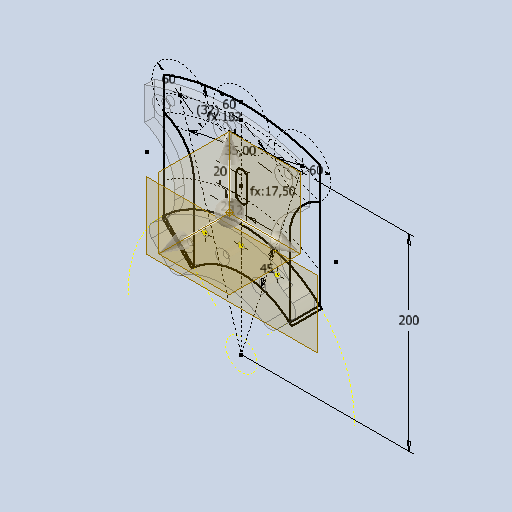
# Autodesk Inventor part: CounterweightFixation_Axis0
Saved by Autodesk Inventor 2024 (Build 280153000, 153)
## iProperties
Created: 2022-10-27
Part Number: CounterweightFixation_Axis0
Material: PMMA-Kunststoff
Document SubType Name: Modeling
Designer: alexw
Mass: 326.548 g
Surface Area: 547.419 cm^2
Volume: 274.872 cm^3
Density: 1.188 g/cm^3
Appearance: Polycarbonat - klar
Author: alexw
Autodesk Inventor part; units mm, degrees
ref_plane "YZ Plane" through (0, 0, 0) normal (1, 0, 0) x (0, 1, 0)
ref_plane "XZ Plane" through (0, 0, 0) normal (0, 1, 0) x (-1, 0, 0)
ref_plane "XY Plane" through (0, 0, 0) normal (0, 0, 1) x (1, 0, 0)
sketch "Skizze1" plane through (0, 0, 0) normal (0, 0, 1) x (1, 0, 0)
  arc A0 (119.8865, -45.2174) -> (-119.8865, -45.2174) centre (0, -40) ccw construction
  arc A1 (53.033, 13.033) -> (-53.033, 13.033) centre (0, -40) ccw construction
  line L0 (53.033, 13.033) -> (84.8528, 44.8528)
  line L1 (26.163, -9.5944) -> (68.5894, 32.832) construction
  line L2 (0, 0) -> (0, 80) construction
  line L3 (-53.033, 13.033) -> (-84.8528, 44.8528)
  arc A2 (53.033, 13.033) -> (-53.033, 13.033) centre (0, -40) ccw
  arc A3 (84.8528, 44.8528) -> (-84.8528, 44.8528) centre (0, -40) ccw
  arc A4 (41.04, 51.2399) -> (35.4967, 53.536) centre (38.2683, 52.388) ccw construction
  arc A5 (-35.4967, 53.536) -> (-41.04, 51.2399) centre (-38.2683, 52.388) ccw construction
  arc A6 (3, 60) -> (-3, 60) centre (0, 60) ccw construction
  line L4 (50.8692, 15.1119) -> (82.705, 46.9476)
  line L5 (-68.5894, 32.832) -> (-26.163, -9.5944) construction
  line L6 (-50.8692, 15.1119) -> (-82.705, 46.9476)
  circle A7 centre (0, -40) radius 16.5 construction
  line L7 (0, -40) -> (0, 160) construction
  arc A8 (82.705, 176.7577) -> (-82.705, 176.7577) centre (0, -40) ccw
  line L8 (82.705, 46.9476) -> (82.705, 176.7577)
  line L9 (-82.705, 46.9476) -> (-82.705, 176.7577)
  arc A9 (82.705, 142.0986) -> (-82.705, 142.0986) centre (0, -40) ccw construction
  line L10 (50.8692, 15.1119) -> (50.8692, 95.7841)
  arc A10 (82.705, 142.0986) -> (50.8692, 95.7841) centre (100.4762, 95.7841) ccw
  arc A11 (82.705, 79.1003) -> (-82.705, 79.1003) centre (0, -40) ccw construction
  line L11 (-50.8692, 15.1119) -> (-50.8692, 95.7841)
  arc A12 (-50.8692, 95.7841) -> (-82.705, 142.0986) centre (-100.4762, 95.7841) ccw
  arc A13 (82.705, 159.5392) -> (-82.705, 159.5392) centre (0, -40) ccw construction
  line L12 (64.9525, 166.0029) -> (0, -40) construction
  line L13 (0, -40) -> (-64.9525, 166.0029) construction
  circle A14 centre (64.9525, 166.0029) radius 30 construction
  circle A15 centre (0, 176) radius 30 construction
  circle A16 centre (-64.9525, 166.0029) radius 30 construction
  line L14 (0, 105) -> (0, 125) construction
  line L15 (6, 105) -> (6, 125)
  line L16 (-6, 125) -> (-6, 105)
  arc A17 (-6, 105) -> (6, 105) centre (0, 105) ccw
  arc A18 (6, 125) -> (-6, 125) centre (0, 125) ccw
  point P0 (0, 192)
  point P1 (-50.8692, 68.6845)
  point P2 (50.8692, 68.6845)
  point P3 (0, 115)
  dimension "d0" = 45
  dimension "d4" = 200
  dimension "d5" = 32
  dimension "d6" = 25
  dimension "d7" = 32
  dimension "d8" = 16
  dimension "d9" = 35
  dimension "d10" = 17.5
  dimension "d11" = 60
  dimension "d12" = 60
  dimension "d13" = 60
  dimension "d32" = 20
  dimension "d33" = 12
  constraints: 37 point on circle, 32 end point, 14 centre point, 11 point on line, 8 coincident, 6 tangent, 4 concentric, 4 symmetric about line, 4 vertical, 2 collinear, 2 line through centre, 2 parallel, 1 midpoint, 1 other
  measures "d0" radial gap between concentric circles of A0 A1
  measures "d4" distance of L7.start L7.end
  measures "d5" distance of point (0, 160) point (0, 192)
  measures "d6" radial gap between concentric circles of A0 A11
  measures "d7" radial gap between concentric circles of A9 A8
  measures "d8" radial gap between concentric circles of A9 A13
  measures "d9" angle of L13 L12
  measures "d10" angle of L12 L7
  measures "d11" diameter of A14
  measures "d12" diameter of A15
  measures "d13" diameter of A16
  measures "d32" distance of L14.start L14.end
  measures "d33" distance between parallel lines of L16 L15
extrude "Extrusion1" add sketch "Skizze1" along normal blind 20 contours L10 A3 L4 | A2 L11 A3 L10 | L6 A3 L11
ref_plane "Arbeitsebene1" through (0, 0, 10) normal (0, 0, 1) x (1, 0, 0)
extrude "Extrusion2" add sketch "Skizze1" against normal blind 10 from surface at 20 contours A3 L11 A12 L9 A8 L8 A10 L10 | A17 L16 A18 L15
hole "Bohrung1" at (38.2683, 52.388, 0) at (0, 60, 0) at (-38.2683, 52.388, 0) direction (0, 0, 1) diameter 6.6 end through all clearance for "Inbusschraube DIN EN ISO 4762" size "M6" standard "DIN"
hole "Bohrung2" at (64.9525, 166.0029, 0) at (0, 176, 0) at (-64.9525, 166.0029, 0) direction (0, 0, 1) diameter 9 end through all clearance for "Inbusschraube DIN EN ISO 4762" size "M8" standard "DIN"
fillet "Rundung1" radius 30 2 edges at (50.8692, 68.6845, 15) (-50.8692, 68.6845, 15)
fillet "Rundung2" radius 10 4 edges at (-82.705, 46.9476, 10) (82.705, 46.9476, 10) (50.8692, 15.1119, 10) (-50.8692, 15.1119, 10)
sketch "Skizze2" plane through (0, 0, 20) normal (0, 0, 1) x (1, 0, 0)
  point P0 (0, 0)
  point P1 (64.9525, 166.0029)
  point P2 (0, 176)
  point P3 (-64.9525, 166.0029)
hole "Bohrung3" at (64.9525, 166.0029, 20) at (0, 176, 20) at (-64.9525, 166.0029, 20) direction (0, 0, -1) diameter 9 end through all countersink diameter 19 countersink angle 90 clearance for "Innensechskant-Senkkopfschraube DIN EN ISO 10642" size "M8" standard "DIN"
sketch "Skizze3" plane through (0, 0, 20) normal (0, 0, 1) x (1, 0, 0)
  point P0 (0, 0)
  point P1 (38.2683, 52.388)
  point P2 (0, 60)
  point P3 (-38.2683, 52.388)
hole "Bohrung4" at (38.2683, 52.388, 20) at (0, 60, 20) at (-38.2683, 52.388, 20) direction (0, 0, -1) diameter 6.6 end through all countersink diameter 14.5 countersink angle 90 clearance for "Innensechskant-Senkkopfschraube DIN EN ISO 10642" size "M6" standard "DIN"
equation "\"d8\" = 0.5 * d7"
equation "\"d10\" = 0.5 * d9"
